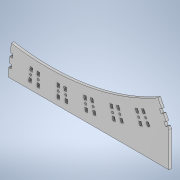
# Autodesk Inventor part: keywell_support-back
Saved by Autodesk Inventor 2020 (Build 240168000, 168)
## iProperties
Created: 2019-06-30
Part Number: keywell_support-back
Material: Acier inoxydable
Document SubType Name: Modeling
Designer: Thibault
Density: 8 g/cm^3
Appearance: Semi-poli
Mass: 13.686 g
Surface Area: 39.9351 cm^2
Volume: 1.71076 cm^3
Author: Thibault
Autodesk Inventor part; units mm, degrees
ref_plane "YZ Plane" through (0, 0, 0) normal (1, 0, 0) x (0, 1, 0)
ref_plane "XZ Plane" through (0, 0, 0) normal (0, 1, 0) x (-1, 0, 0)
ref_plane "XY Plane" through (0, 0, 0) normal (0, 0, 1) x (1, 0, 0)
sketch "anchor" plane through (0, 0, 0) normal (0, 0, 1) x (1, 0, 0)
  circle A0 centre (-8.6489, 1.6726) radius 0.85
  line L0 (-7.6489, 7.1726) -> (-9.6489, 7.1726)
  line L1 (-9.6489, 7.1726) -> (-9.6489, 4.1726)
  line L2 (-9.6489, 4.1726) -> (-7.6489, 4.1726)
  line L3 (-7.6489, 4.1726) -> (-7.6489, 7.1726)
  line L4 (-7.6489, -0.8274) -> (-9.6489, -0.8274)
  line L5 (-9.6489, -0.8274) -> (-9.6489, -3.8274)
  line L6 (-9.6489, -3.8274) -> (-7.6489, -3.8274)
  line L7 (-7.6489, -3.8274) -> (-7.6489, -0.8274)
  circle A1 centre (7.3511, 1.6726) radius 0.85
  line L8 (6.3511, 7.1726) -> (8.3511, 7.1726)
  line L9 (8.3511, 7.1726) -> (8.3511, 4.1726)
  line L10 (8.3511, 4.1726) -> (6.3511, 4.1726)
  line L11 (6.3511, 4.1726) -> (6.3511, 7.1726)
  line L12 (6.3511, -0.8274) -> (8.3511, -0.8274)
  line L13 (8.3511, -0.8274) -> (8.3511, -3.8274)
  line L14 (8.3511, -3.8274) -> (6.3511, -3.8274)
  line L15 (6.3511, -3.8274) -> (6.3511, -0.8274)
  line L16 (-9.6489, 4.1726) -> (-7.6489, -0.8274) construction
  line L17 (-9.6489, -0.8274) -> (-7.6489, 4.1726) construction
  line L18 (6.3511, 4.1726) -> (8.3511, -0.8274) construction
  line L19 (6.3511, -0.8274) -> (8.3511, 4.1726) construction
  line L20 (-8.6489, 1.6726) -> (-0.6489, 1.6726) construction
  line L21 (-0.6489, 1.6726) -> (7.3511, 1.6726) construction
  point P0 (-0.0015, -0.1178)
  dimension "d18" = 1.7
  dimension "d23" = 3
  dimension "d24" = 2
  dimension "d25" = 3
  dimension "d122" = 5
  dimension "d123" = 1.7
  dimension "d124" = 2
  dimension "d125" = 2
  dimension "d127" = 2
  dimension "d128" = 14
  measures "d18" diameter of A0
  measures "d23" distance of L1.end L0.end
  measures "d24" distance of L6.end L5.end
  measures "d25" distance of L5.end L4.end
  measures "d122" distance of L4.end L1.end
  measures "d123" diameter of A1
  measures "d124" distance of L14.start L14.end
  measures "d125" distance of L8.start L8.end
  measures "d127" distance of L0.start L0.end
  measures "d128" distance between parallel lines of L11 L3
sketch "anchor_external" plane through (0, 0, 0) normal (0, 0, 1) x (1, 0, 0)
  circle A0 centre (-9.0028, -0.9968) radius 0.85
  line L0 (-8.0028, 4.5032) -> (-10.0028, 4.5032)
  line L1 (-10.0028, 4.5032) -> (-10.0028, 1.5032)
  line L2 (-10.0028, 1.5032) -> (-8.0028, 1.5032)
  line L3 (-8.0028, 1.5032) -> (-8.0028, 4.5032)
  line L4 (-8.0028, -3.4968) -> (-10.0028, -3.4968)
  line L5 (-10.0028, -3.4968) -> (-10.0028, -6.4968)
  line L6 (-10.0028, -6.4968) -> (-8.0028, -6.4968)
  line L7 (-8.0028, -6.4968) -> (-8.0028, -3.4968)
  line L8 (7.9972, 1.5032) -> (5.9972, 1.5032)
  line L9 (5.9972, -3.4968) -> (7.9972, -3.4968)
  line L10 (5.9972, 4.5032) -> (7.9972, 4.5032)
  line L11 (7.9972, -6.4968) -> (5.9972, -6.4968)
  line L12 (5.9972, -6.4968) -> (5.9972, -3.4968)
  line L13 (1.4567, -0.9968) -> (-3, -0.9968) construction
  line L14 (5.9972, 1.5032) -> (5.9972, 4.5032)
  line L15 (7.9972, 1.5032) -> (7.9972, -3.4968)
  line L16 (-10.0028, 1.5032) -> (-8.0028, -3.4968) construction
  line L17 (-10.0028, -3.4968) -> (-8.0028, 1.5032) construction
  point P0 (-0.3208, -0.9968)
  point P1 (-1.0028, -0.9968)
  dimension "d80" = 1.7
  dimension "d83" = 3
  dimension "d84" = 2
  dimension "d85" = 3
  dimension "d132" = 7
  dimension "d133" = 7
  dimension "d158" = 2
  dimension "d159" = 5
  measures "d80" diameter of A0
  measures "d83" distance of L1.end L0.end
  measures "d84" distance of L6.end L5.end
  measures "d85" distance of L5.end L4.end
  measures "d132" horizontal distance of L8.end point (-1.003, -0.997)
  measures "d133" distance from line of L3 point (-1.003, -0.997)
  measures "d158" distance of L11.start L11.end
  measures "d159" distance between parallel lines of L4 L2
sketch "Esquisse2" plane through (0, 0, 0) normal (0, 0, 1) x (1, 0, 0)
  circle A0 centre (0, 0) radius 190 construction
  arc A1 (-29.3574, -175.5624) -> (87.6328, -154.9338) centre (0, 0) ccw
  line L0 (96.4644, -200.2468) -> (-31.6231, -200.2468)
  line L1 (-30.13, -182.2455) -> (-29.3574, -175.5624)
  line L2 (-31.3934, -193.1727) -> (-31.6231, -195.1595)
  line L3 (90.6446, -160.9497) -> (87.6328, -154.9338)
  line L4 (95.5691, -170.7858) -> (96.4644, -172.5742)
  line L5 (30.4039, -182.2) -> (33.7457, -181.6108) construction
  line L6 (49.6599, -108.847) -> (49.6599, -114.6161) construction
  line L7 (96.4644, -172.5742) -> (96.4644, -200.2468)
  line L8 (-31.6231, -195.1595) -> (-31.6231, -200.2468)
  circle A2 centre (-7.8572, -190.006) radius 0.85
  line L9 (-6.8613, -184.5052) -> (-8.8613, -184.5067)
  line L10 (-8.8613, -184.5067) -> (-8.8591, -187.5067)
  line L11 (-8.8591, -187.5067) -> (-6.8591, -187.5052)
  line L12 (-6.8591, -187.5052) -> (-6.8613, -184.5052)
  line L13 (-6.8553, -192.5052) -> (-8.8553, -192.5067)
  line L14 (-8.8553, -192.5067) -> (-8.8531, -195.5067)
  line L15 (-8.8531, -195.5067) -> (-6.8531, -195.5052)
  line L16 (-6.8531, -195.5052) -> (-6.8553, -192.5052)
  circle A3 centre (8.1428, -189.9939) radius 0.85
  line L17 (7.1387, -184.4947) -> (9.1387, -184.4932)
  line L18 (9.1387, -184.4932) -> (9.1409, -187.4932)
  line L19 (9.1409, -187.4932) -> (7.1409, -187.4947)
  line L20 (7.1409, -187.4947) -> (7.1387, -184.4947)
  line L21 (7.1447, -192.4947) -> (9.1447, -192.4932)
  line L22 (9.1447, -192.4932) -> (9.1469, -195.4932)
  line L23 (9.1469, -195.4932) -> (7.1469, -195.4947)
  line L24 (7.1469, -195.4947) -> (7.1447, -192.4947)
  line L25 (-8.8591, -187.5067) -> (-6.8553, -192.5052) construction
  line L26 (-8.8553, -192.5067) -> (-6.8591, -187.5052) construction
  line L27 (7.1409, -187.4947) -> (9.1447, -192.4932) construction
  line L28 (7.1447, -192.4947) -> (9.1409, -187.4932) construction
  line L29 (-7.8572, -190.006) -> (0.1428, -189.9999) construction
  line L30 (0.1428, -189.9999) -> (8.1428, -189.9939) construction
  circle A4 centre (57.33, -181.3209) radius 0.85
  line L31 (56.3928, -175.8099) -> (54.5129, -176.4925)
  line L32 (54.5129, -176.4925) -> (55.5368, -179.3123)
  line L33 (55.5368, -179.3123) -> (57.4167, -178.6297)
  line L34 (57.4167, -178.6297) -> (56.3928, -175.8099)
  line L35 (59.1233, -183.3295) -> (57.2434, -184.0121)
  line L36 (57.2434, -184.0121) -> (58.2673, -186.8319)
  line L37 (58.2673, -186.8319) -> (60.1472, -186.1493)
  line L38 (60.1472, -186.1493) -> (59.1233, -183.3295)
  circle A5 centre (72.3692, -175.8599) radius 0.85
  line L39 (69.552, -171.0315) -> (71.4319, -170.3488)
  line L40 (71.4319, -170.3488) -> (72.4559, -173.1687)
  line L41 (72.4559, -173.1687) -> (70.576, -173.8513)
  line L42 (70.576, -173.8513) -> (69.552, -171.0315)
  line L43 (72.2826, -178.5511) -> (74.1625, -177.8684)
  line L44 (74.1625, -177.8684) -> (75.1864, -180.6883)
  line L45 (75.1864, -180.6883) -> (73.3065, -181.3709)
  line L46 (73.3065, -181.3709) -> (72.2826, -178.5511)
  line L47 (55.5368, -179.3123) -> (59.1233, -183.3295) construction
  line L48 (57.2434, -184.0121) -> (57.4167, -178.6297) construction
  line L49 (70.576, -173.8513) -> (74.1625, -177.8684) construction
  line L50 (72.2826, -178.5511) -> (72.4559, -173.1687) construction
  line L51 (57.33, -181.3209) -> (64.8496, -178.5904) construction
  line L52 (64.8496, -178.5904) -> (72.3692, -175.8599) construction
  circle A6 centre (35.9859, -186.7325) radius 0.85
  line L53 (35.6919, -181.15) -> (33.7457, -181.6108)
  line L54 (33.7457, -181.6108) -> (34.4368, -184.5301)
  line L55 (34.4368, -184.5301) -> (36.3831, -184.0693)
  line L56 (36.3831, -184.0693) -> (35.6919, -181.15)
  line L57 (37.5349, -188.9349) -> (35.5887, -189.3956)
  line L58 (35.5887, -189.3956) -> (36.2798, -192.3149)
  line L59 (36.2798, -192.3149) -> (38.226, -191.8542)
  line L60 (38.226, -191.8542) -> (37.5349, -188.9349)
  circle A7 centre (51.5555, -183.0465) radius 0.85
  line L61 (49.3154, -177.9248) -> (51.2616, -177.4641)
  line L62 (51.2616, -177.4641) -> (51.9527, -180.3834)
  line L63 (51.9527, -180.3834) -> (50.0065, -180.8441)
  line L64 (50.0065, -180.8441) -> (49.3154, -177.9248)
  line L65 (51.1583, -185.7096) -> (53.1046, -185.2489)
  line L66 (53.1046, -185.2489) -> (53.7957, -188.1682)
  line L67 (53.7957, -188.1682) -> (51.8495, -188.629)
  line L68 (51.8495, -188.629) -> (51.1583, -185.7096)
  line L69 (34.4368, -184.5301) -> (37.5349, -188.9349) construction
  line L70 (35.5887, -189.3956) -> (36.3831, -184.0693) construction
  line L71 (50.0065, -180.8441) -> (53.1046, -185.2489) construction
  line L72 (51.1583, -185.7096) -> (51.9527, -180.3834) construction
  line L73 (35.9859, -186.7325) -> (43.7707, -184.8895) construction
  line L74 (43.7707, -184.8895) -> (51.5555, -183.0465) construction
  circle A8 centre (-13.8742, -189.6616) radius 0.85
  line L75 (-15.4992, -195.0103) -> (-13.5125, -195.24)
  line L76 (-13.5125, -195.24) -> (-13.1679, -192.2599)
  line L77 (-13.1679, -192.2599) -> (-15.1547, -192.0302)
  line L78 (-15.1547, -192.0302) -> (-15.4992, -195.0103)
  line L79 (-14.5805, -187.0633) -> (-12.5937, -187.2929)
  line L80 (-12.5937, -187.2929) -> (-12.2491, -184.3128)
  line L81 (-12.2491, -184.3128) -> (-14.2359, -184.0831)
  line L82 (-14.2359, -184.0831) -> (-14.5805, -187.0633)
  line L83 (-31.0488, -190.1926) -> (-29.0621, -190.4223)
  line L84 (-28.4878, -185.4554) -> (-30.4746, -185.2257)
  line L85 (-29.4066, -193.4024) -> (-31.3934, -193.1727)
  line L86 (-30.13, -182.2455) -> (-28.1433, -182.4752)
  line L87 (-28.1433, -182.4752) -> (-28.4878, -185.4554)
  line L88 (-24.2645, -188.4603) -> (-19.8373, -188.9721) construction
  line L89 (-29.0621, -190.4223) -> (-29.4066, -193.4024)
  line L90 (-31.0488, -190.1926) -> (-30.4746, -185.2257)
  line L91 (-13.1679, -192.2599) -> (-14.5805, -187.0633) construction
  line L92 (-12.5937, -187.2929) -> (-15.1547, -192.0302) construction
  circle A9 centre (77.9056, -173.4783) radius 0.85
  line L93 (76.3375, -168.1126) -> (74.5491, -169.0079)
  line L94 (74.5491, -169.0079) -> (75.8922, -171.6905)
  line L95 (75.8922, -171.6905) -> (77.6805, -170.7951)
  line L96 (77.6805, -170.7951) -> (76.3375, -168.1126)
  line L97 (79.9189, -175.2661) -> (78.1306, -176.1615)
  line L98 (78.1306, -176.1615) -> (79.4736, -178.8441)
  line L99 (79.4736, -178.8441) -> (81.262, -177.9487)
  line L100 (81.262, -177.9487) -> (79.9189, -175.2661)
  line L101 (91.9877, -163.6323) -> (90.1993, -164.5276)
  line L102 (92.4377, -168.9986) -> (94.226, -168.1032)
  line L103 (88.8562, -161.8451) -> (90.6446, -160.9497)
  line L104 (95.5691, -170.7858) -> (93.7807, -171.6812)
  line L105 (93.7807, -171.6812) -> (92.4377, -168.9986)
  line L106 (87.2584, -168.7958) -> (83.2732, -170.791) construction
  line L107 (90.1993, -164.5276) -> (88.8562, -161.8451)
  line L108 (91.9877, -163.6323) -> (94.226, -168.1032)
  line L109 (75.8922, -171.6905) -> (79.9189, -175.2661) construction
  line L110 (78.1306, -176.1615) -> (77.6805, -170.7951) construction
  circle A10 centre (14.1593, -189.6405) radius 0.85
  line L111 (14.5126, -184.0615) -> (12.5262, -184.2942)
  line L112 (12.5262, -184.2942) -> (12.8752, -187.2738)
  line L113 (12.8752, -187.2738) -> (14.8616, -187.0411)
  line L114 (14.8616, -187.0411) -> (14.5126, -184.0615)
  line L115 (15.4433, -192.0072) -> (13.4569, -192.2399)
  line L116 (13.4569, -192.2399) -> (13.8059, -195.2195)
  line L117 (13.8059, -195.2195) -> (15.7923, -194.9868)
  line L118 (15.7923, -194.9868) -> (15.4433, -192.0072)
  circle A11 centre (30.0506, -187.779) radius 0.85
  line L119 (28.4175, -182.4327) -> (30.4039, -182.2)
  line L120 (30.4039, -182.2) -> (30.753, -185.1797)
  line L121 (30.753, -185.1797) -> (28.7665, -185.4123)
  line L122 (28.7665, -185.4123) -> (28.4175, -182.4327)
  line L123 (29.3482, -190.3784) -> (31.3347, -190.1457)
  line L124 (31.3347, -190.1457) -> (31.6837, -193.1253)
  line L125 (31.6837, -193.1253) -> (29.6973, -193.358)
  line L126 (29.6973, -193.358) -> (29.3482, -190.3784)
  line L127 (12.8752, -187.2738) -> (15.4433, -192.0072) construction
  line L128 (13.4569, -192.2399) -> (14.8616, -187.0411) construction
  line L129 (28.7665, -185.4123) -> (31.3347, -190.1457) construction
  line L130 (29.3482, -190.3784) -> (30.753, -185.1797) construction
  line L131 (14.1593, -189.6405) -> (22.1049, -188.7098) construction
  line L132 (22.1049, -188.7098) -> (30.0506, -187.779) construction
  point P0 (-31.3934, -193.1727)
  point P1 (-30.13, -182.2455)
  point P2 (95.5691, -170.7858)
  point P3 (61.9481, -201.7719)
  dimension "d32" = 2
  dimension "d130" = 22
  dimension "d131" = 22
  dimension "d134" = 22
  dimension "d135" = 22
  dimension "distance" = 22
  dimension "radius" = 380
  dimension "d73" = 178
  dimension "angle" = 80
  dimension "d154" = 2
  dimension "d157" = 2
  constraints: 19 end point, 3 vertical, 2 centre point, 2 point on circle, 1 coincident, 23 other
  measures "radius" diameter of A0
  measures "d73" radius of A1
  measures "angle" angle of L5 L6
  measures "d154" distance of L4.start L4.end
  measures "d157" distance of L2.start L2.end
extrude "Base" add sketch "Esquisse2" along normal blind 2
sketch "Esquisse5" plane through (0, 0, 2) normal (0, 0, 1) x (1, 0, 0)
  line L0 (48.8123, -108.0562) -> (186.217, -108.0562)
  line L1 (186.217, -108.0562) -> (186.217, -259.9576)
  line L2 (75.869, -182.5682) -> (75.1864, -180.6883)
  line L3 (69.552, -171.0315) -> (71.4319, -170.3488) projected
  line L4 (70.576, -173.8513) -> (69.552, -171.0315) projected
  line L5 (72.4559, -173.1687) -> (70.576, -173.8513) projected
  line L6 (72.2826, -178.5511) -> (74.1625, -177.8684) projected
  line L7 (73.3065, -181.3709) -> (72.2826, -178.5511) projected
  line L8 (75.1864, -180.6883) -> (73.3065, -181.3709) projected
  line L9 (48.8123, -108.0562) -> (71.4319, -170.3488)
  line L10 (71.4319, -170.3488) -> (72.4559, -173.1687) projected
  line L11 (72.4559, -173.1687) -> (74.1625, -177.8684)
  line L12 (75.869, -182.5682) -> (75.869, -259.9576)
  line L13 (75.869, -259.9576) -> (186.217, -259.9576)
  point P0 (0, 0)
  point P1 (77.6805, -170.7951)
  point P2 (79.9189, -175.2661)
  dimension "d155" = 2
  constraints: 14 end point, 3 perpendicular, 1 collinear, 1 horizontal, 1 vertical
  measures "d155" distance of L2.start L2.end
extrude "Front: substract" [suppressed]
sketch "Esquisse6" plane through (0, 0, 2) normal (0, 0, 1) x (1, 0, 0)
  line L0 (68.8371, -174.4827) -> (72.4559, -173.1687)
  line L1 (70.5437, -179.1825) -> (74.1625, -177.8684)
  line L2 (72.4559, -173.1687) -> (70.576, -173.8513) projected
  line L3 (72.2826, -178.5511) -> (74.1625, -177.8684) projected
  line L4 (68.8371, -174.4827) -> (70.5437, -179.1825)
  line L5 (74.1625, -177.8684) -> (72.4559, -173.1687) projected
  line L6 (72.4559, -173.1687) -> (74.1625, -177.8684)
  circle A0 centre (72.3692, -175.8599) radius 0.85 projected
  point P0 (0, 0)
  point P1 (73.1682, -175.5698)
  point P2 (73.1682, -175.5698)
  point P3 (71.5703, -176.15)
  point P4 (72.2826, -178.5511)
  point P5 (70.7469, -175.7787)
  point P6 (70.576, -173.8513)
  dimension "d146" = 2
  dimension "d152" = 2
  constraints: 6 end point, 2 coincident, 2 collinear, 5 other
  measures "d146" distance from line of L4 point (71.57, -176.15)
  measures "d152" distance edge to line of A0 L4
extrude "Front: fill" [suppressed]
sketch "Esquisse7" plane through (0, 0, 2) normal (0, 0, 1) x (1, 0, 0)
  line L0 (75.6984, -182.0982) -> (57.2981, -131.4254)
  line L1 (74.1625, -177.8684) -> (75.1864, -180.6883) projected
  line L2 (-105.9622, -264.9128) -> (-94.3872, -119.3625)
  line L3 (-94.3872, -119.3625) -> (57.2981, -131.4254)
  line L4 (75.6984, -182.0982) -> (75.6984, -264.9128)
  line L5 (75.6984, -264.9128) -> (-105.9622, -264.9128)
  point P0 (0, 0)
  dimension "d156" = 1.5
  constraints: 10 end point, 2 perpendicular, 1 collinear, 1 vertical
  measures "d156" distance of L0.start L1.end
extrude "Front r6: substract" [suppressed]
sketch "Esquisse8" plane through (0, 0, 2) normal (0, 0, 1) x (1, 0, 0)
  line L0 (69.552, -171.0315) -> (71.4319, -170.3488) projected
  line L1 (70.576, -173.8513) -> (69.552, -171.0315) projected
  line L2 (72.4559, -173.1687) -> (70.576, -173.8513) projected
  line L3 (71.4319, -170.3488) -> (72.4559, -173.1687) projected
  line L4 (72.2826, -178.5511) -> (74.1625, -177.8684) projected
  line L5 (73.3065, -181.3709) -> (72.2826, -178.5511) projected
  line L6 (75.1864, -180.6883) -> (73.3065, -181.3709) projected
  line L7 (74.1625, -177.8684) -> (75.1864, -180.6883) projected
  point P0 (0, 0)
extrude "Front r6: fill" [suppressed]
